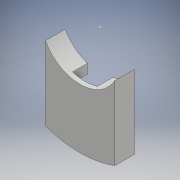
# Autodesk Inventor part: piston_mount_ring_full
Saved by Autodesk Inventor 2018 (Build 220112000, 112)
## iProperties
Created: 2026-05-03
Part Number: piston_mount_ring_full
Material: Generic
Document SubType Name: Modeling
Designer: neo
Density: 1 g/cm^3
Appearance: Default
Author: neo
Autodesk Inventor part; units mm, degrees
ref_plane "YZ Plane" through (0, 0, 0) normal (1, 0, 0) x (0, 1, 0)
ref_plane "XZ Plane" through (0, 0, 0) normal (0, 1, 0) x (-1, 0, 0)
ref_plane "XY Plane" through (0, 0, 0) normal (0, 0, 1) x (1, 0, 0)
sketch "Sketch1" plane through (0, 0, 0) normal (0, 1, 0) x (-1, 0, 0)
  circle A0 centre (0, 0) radius 80
  circle A1 centre (0, 0) radius 200
  dimension "d0" = 400
  dimension "d1" = 120
  dimension "d2" = 160
  constraints: 2 centre point, 2 coincident
  measures "d0" diameter of A1
  measures "d1" radial gap between concentric circles of A1 A0
  measures "d2" diameter of A0
extrude "Extrusion1" add sketch "Sketch1" along normal blind 40
sketch "Sketch2" plane through (0, 40, 0) normal (0, 1, 0) x (1, 0, 0)
  point P0 (0, 0)
sketch "Sketch3" plane through (0, 40, 0) normal (0, 1, 0) x (1, 0, 0)
  line L0 (0, 0) -> (0, 239.087)
  line L1 (50, 40.8178) -> (-50, 40.8178)
  line L2 (-50, 40.8178) -> (-50, 200)
  line L3 (-50, 200) -> (50, 200)
  line L4 (50, 200) -> (50, 40.8178)
  circle A0 centre (0, 0) radius 200 construction
  dimension "d5" = 100
  constraints: 10 end point, 2 parallel, 1 horizontal, 1 perpendicular, 1 tangent, 1 vertical, 1 other
  measures "d5" distance of L1.start L1.end
extrude "Extrusion2" cut sketch "Sketch3" against normal blind 30
sketch "Sketch4" plane through (0, 10, 0) normal (0, 1, 0) x (1, 0, 0)
  arc A0 (50, 62.45) -> (-50, 62.45) centre (0, 0) ccw construction
  line L0 (50, 193.6492) -> (50, 62.45) construction
  arc A1 (50, 193.6492) -> (-50, 193.6492) centre (0, 0) ccw construction
  line L1 (-50, 62.45) -> (-50, 193.6492) construction
  circle A2 centre (0, 0) radius 80 construction
  line L2 (0, 80) -> (0, 200)
  circle A3 centre (0, 0) radius 200 construction
  arc A4 (50, 62.45) -> (25.25, 75.9107) centre (0, 0) ccw
  line L3 (50, 62.45) -> (50, 95)
  line L4 (50, 193.6492) -> (50, 62.45) projected
  line L5 (31.55, 95) -> (31.55, 87)
  line L6 (31.55, 87) -> (28.45, 87)
  line L7 (28.45, 87) -> (28.45, 95)
  line L8 (28.45, 95) -> (25.25, 95)
  line L9 (25.25, 95) -> (25.25, 75.9107)
  line L10 (31.55, 95) -> (50, 95)
  arc A5 (50, 62.45) -> (-50, 62.45) centre (0, 0) ccw construction
  line L11 (-50, 193.6492) -> (-50, 62.45) construction
  circle A6 centre (0, 0) radius 80 construction
  arc A7 (-25.25, 75.9107) -> (-50, 62.45) centre (0, 0) ccw
  line L12 (-50, 62.45) -> (-50, 95)
  line L13 (-50, 193.6492) -> (-50, 62.45)
  line L14 (-31.55, 95) -> (-31.55, 87)
  line L15 (-31.55, 87) -> (-28.45, 87)
  line L16 (-28.45, 87) -> (-28.45, 95)
  line L17 (-28.45, 95) -> (-25.25, 95)
  line L18 (-25.25, 95) -> (-25.25, 75.9107)
  line L19 (-31.55, 95) -> (-50, 95)
  arc A8 (50, 193.6492) -> (25.25, 198.3997) centre (0, 0) ccw
  line L20 (50, 193.6492) -> (50, 185)
  line L21 (31.55, 185) -> (31.55, 193)
  line L22 (31.55, 193) -> (28.45, 193)
  line L23 (28.45, 193) -> (28.45, 185)
  line L24 (25.25, 185) -> (25.25, 198.3997)
  line L25 (31.55, 185) -> (50, 185)
  line L26 (28.45, 185) -> (25.25, 185)
  arc A9 (-25.25, 198.3997) -> (-50, 193.6492) centre (0, 0) ccw
  line L27 (-50, 193.6492) -> (-50, 185)
  line L28 (-31.55, 185) -> (-31.55, 193)
  line L29 (-31.55, 193) -> (-28.45, 193)
  line L30 (-28.45, 193) -> (-28.45, 185)
  line L31 (-25.25, 185) -> (-25.25, 198.3997)
  line L32 (-31.55, 185) -> (-50, 185)
  line L33 (-28.45, 185) -> (-25.25, 185)
  line L34 (30, 87) -> (30, 88.6498)
  line L35 (-30, 87) -> (-30, 88.6498)
  point P0 (25.25, 75.7218)
  point P1 (-25.25, 75.7218)
  point P2 (-39.9698, 182.9054)
  point P3 (26.85, 185)
  point P4 (31.55, 189)
  dimension "d11" = 90
  dimension "d12" = 3.1
  dimension "d13" = 3.2
  dimension "d14" = 60
  dimension "d15" = 8
  dimension "d16" = 95
  dimension "d17" = 8
  constraints: 66 end point, 17 point on circle, 17 symmetric about line, 7 point on line, 6 centre point, 5 perpendicular, 4 midpoint, 3 collinear, 3 horizontal, 3 vertical, 2 coincident, 2 parallel, 1 concentric, 4 other
  measures "d11" distance between parallel lines of L10 L25
  measures "d12" distance between parallel lines of L7 L5
  measures "d13" distance between parallel lines of L24 L23
  measures "d14" distance between parallel lines of L35 L34
  measures "d15" distance between parallel lines of L10 L6
  measures "d16" distance from line of A0.centre L10
  measures "d17" distance from line of L25 L21.end
extrude "Extrusion3" add sketch "Sketch4" along normal up to surface (30 mm away)
sketch "Sketch5" plane through (0, 10, 0) normal (0, 1, 0) x (1, 0, 0)
  line L0 (31.55, 87) -> (31.55, 95) projected
  line L1 (28.45, 95) -> (28.45, 87) projected
  line L2 (31.55, 87) -> (28.45, 87)
  line L3 (28.45, 87) -> (28.45, 95)
  line L4 (28.45, 95) -> (31.55, 95)
  line L5 (31.55, 95) -> (31.55, 87)
  line L6 (-50, 95) -> (-31.55, 95) projected
  line L7 (-28.4346, 87) -> (-31.55, 87)
  line L8 (-31.55, 87) -> (-31.55, 95)
  line L9 (-31.55, 95) -> (-28.4346, 95)
  line L10 (-28.4346, 95) -> (-28.4346, 87)
  line L11 (31.55, 185) -> (31.55, 193) projected
  line L12 (28.45, 193) -> (28.45, 185) projected
  line L13 (31.55, 185) -> (28.45, 185)
  line L14 (28.45, 185) -> (28.45, 193)
  line L15 (28.45, 193) -> (31.55, 193)
  line L16 (31.55, 193) -> (31.55, 185)
  line L17 (-31.55, 193) -> (-31.55, 185) projected
  line L18 (-28.4346, 185) -> (-31.55, 185)
  line L19 (-31.55, 185) -> (-31.55, 193)
  line L20 (-31.55, 193) -> (-28.4346, 193)
  line L21 (-28.4346, 193) -> (-28.4346, 185)
  point P0 (0, 0)
  constraints: 32 end point, 8 parallel, 4 horizontal, 4 perpendicular, 2 point on line
extrude "Extrusion4" add sketch "Sketch5" along normal blind 15
sketch "Sketch9" plane through (0, 40, 0) normal (0, 1, 0) x (1, 0, 0)
  line L0 (0, 0) -> (0, 302.2728)
  line L1 (70, 3.2747) -> (70, 266.6364)
  line L2 (-70, 3.2747) -> (-70, 266.6364)
  arc A0 (-70, 3.2747) -> (70, 3.2747) centre (0, 0) ccw
  arc A1 (-70, 266.6364) -> (70, 266.6364) centre (0, 0) ccw
  dimension "d34" = 140
  constraints: 6 end point, 4 point on circle, 2 centre point, 2 coincident, 2 symmetric about line, 2 vertical
  measures "d34" distance between parallel lines of L1 L2
extrude "Extrusion8" cut sketch "Sketch9" against normal through all
body "Solid1"
